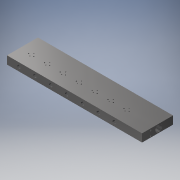
# Autodesk Inventor part: Ventilblock_4
Saved by Autodesk Inventor 2018 (Build 220112000, 112)
## iProperties
Created: 2011-11-24
Part Number: Ventilblock_4
Document SubType Name: Modeling
Designer: Neef
Density: 8 g/cm^3
Material: Stainless Steel
Appearance: Semi-Polished
Author: Neef
Autodesk Inventor part; units mm, degrees
ref_plane "YZ Plane" through (0, 0, 0) normal (1, 0, 0) x (0, 1, 0)
ref_plane "XZ Plane" through (0, 0, 0) normal (0, 1, 0) x (-1, 0, 0)
ref_plane "XY Plane" through (0, 0, 0) normal (0, 0, 1) x (1, 0, 0)
sketch "Skizze1" plane through (0, 0, 0) normal (0, 0, 1) x (1, 0, 0)
  line L0 (-85, 19.5) -> (85, 19.5)
  line L1 (85, 19.5) -> (85, -19.5)
  line L2 (85, -19.5) -> (-85, -19.5)
  line L3 (-85, -19.5) -> (-85, 19.5)
  line L4 (0, 27.3) -> (0, -27.3) projected
  line L5 (-119, 0) -> (119, 0) projected
  point P0 (0, 19.5)
  point P1 (85, 0)
  dimension "d0" = 39
  dimension "d1" = 170
  constraints: 8 end point, 2 midpoint, 2 parallel, 2 point on line, 1 horizontal, 1 perpendicular
  measures "d0" distance of L0.end L1.end
  measures "d1" distance of L0.start L0.end
extrude "Extrusion1" add sketch "Skizze1" along normal blind 10
sketch "Skizze2" plane through (0, 0, 10) normal (0, 0, 1) x (1, 0, 0)
  line L0 (-85, 19.5) -> (85, 19.5) projected
  line L1 (-85, -19.5) -> (-85, 19.5) projected
  line L2 (-75, 17.5) -> (-65, 17.5) construction
  line L3 (-65, 17.5) -> (-65, -9.5) construction
  line L4 (-65, -9.5) -> (-75, -9.5) construction
  line L5 (-75, -9.5) -> (-75, 17.5) construction
  line L6 (-70, -9.5) -> (-70, -1.8624) construction
  point P0 (-70, -0.7)
  point P1 (-70, -5.7)
  dimension "d6" = 10
  dimension "d7" = 27
  dimension "d8" = 5
  dimension "d9" = 10
  dimension "d10" = 3.8
  dimension "d11" = 2
  dimension "d12" = 5
  constraints: 10 end point, 2 parallel, 2 point on line, 1 horizontal, 1 midpoint, 1 perpendicular, 1 vertical
  measures "d6" distance of L2.start L2.end
  measures "d7" distance of L4.end L2.start
  measures "d8" distance between parallel lines of L3 L6
  measures "d9" distance between parallel lines of L5 L1
  measures "d10" distance from line of point (-70, -5.7) L4
  measures "d11" distance between parallel lines of L0 L2
  measures "d12" distance of point (-70, -5.7) point (-70, -0.7)
hole "Bohrung1" at (-70, -0.7, 10) at (-70, -5.7, 10) direction (0, 0, -1) diameter 1.2 depth 5 tip angle 118
sketch "Skizze3" plane through (0, 0, 10) normal (0, 0, 1) x (1, 0, 0)
  circle A0 centre (-70, -5.7) radius 0.6 projected
  circle A1 centre (-70, -0.7) radius 0.6 projected
  point P0 (-73.25, -4)
  point P1 (-66.75, -4)
  dimension "d20" = 3.25
  dimension "d21" = 3.25
  dimension "d22" = 1.7
  dimension "d23" = 1.7
  measures "d20" horizontal distance of A1.centre point (-66.75, -4)
  measures "d21" horizontal distance of A1.centre point (-73.25, -4)
  measures "d22" vertical distance of point (-66.75, -4) A0.centre
  measures "d23" vertical distance of A0.centre point (-73.25, -4)
hole "Bohrung2" at (-73.25, -4, 10) at (-66.75, -4, 10) direction (0, 0, -1) diameter 1.221 depth 7 tip angle 118 thread size "M1.6x0.35" class "6H" standard "ISO Metric profile"
pattern_linear "Rechteckige Anordnung1" count 7 spacing 20 along (1, 0, 0) of "Bohrung1", "Bohrung2"
sketch "Skizze5" plane through (-85, -19.5, 0) normal (0, -1, 0) x (1, 0, 0)
  line L0 (170, 10) -> (0, 10) projected
  line L1 (0, 0) -> (0, 10) projected
  line L2 (15.6, 5) -> (15.6, 10) projected
  line L3 (15.6, 5) -> (14.4, 5) projected
  line L4 (14.4, 5) -> (14.4, 10) projected
  point P0 (15, 5)
  dimension "d53" = 15
  dimension "d54" = 5
  constraints: 1 midpoint
  measures "d53" distance from line of L1 point (15, 5)
  measures "d54" distance from line of L0 point (15, 5)
hole "Bohrung5" at (-70, -19.5, 5) direction (0, 1, 0) diameter 2 depth 14 tip angle 118
hole "Bohrung6" at (-70, -19.5, 5) direction (0, 1, 0) diameter 4.134 depth 7 tip angle 118 thread size "M5x0.8" class "6H" standard "ISO Metric profile"
pattern_linear "Rechteckige Anordnung2" count 7 spacing 20 along (1, 0, 0) of "Bohrung5", "Bohrung6"
sketch "Skizze8" plane through (-85, -19.5, 0) normal (-1, 0, 0) x (0, 0, 1)
  line L0 (10, 0) -> (10, 39) projected
  line L1 (0, 39) -> (10, 39) projected
  line L2 (0, 0) -> (0, 39) projected
  point P0 (0, 19.5)
  point P1 (2, 11)
  point P2 (8, 11)
  dimension "d145" = 28
  dimension "d146" = 28
  dimension "d147" = 2
  dimension "d148" = 2
  measures "d145" distance from line of L1 point (8, 11)
  measures "d146" distance from line of L1 point (2, 11)
  measures "d147" distance from line of L0 point (8, 11)
  measures "d148" distance from line of L2 point (2, 11)
hole "Bohrung14" at (-85, -8.5, 2) at (-85, -8.5, 8) direction (1, 0, 0) diameter 2.459 depth 12 tip angle 118 thread size "M3x0.5" class "6H" standard "ISO Metric profile"
sketch "Skizze9" plane through (85, -19.5, 0) normal (1, 0, 0) x (0, 0, -1)
  circle A0 centre (-8, 11) radius 1.2295 projected
  circle A1 centre (-2, 11) radius 1.2295 projected
  point P0 (0, 19.5)
  constraints: 2 coincident
hole "Bohrung15" at (85, -8.5, 8) at (85, -8.5, 2) direction (-1, 0, 0) diameter 2.459 depth 12 tip angle 118 thread size "M3x0.5" class "6H" standard "ISO Metric profile"
sketch "Skizze10" plane through (85, -19.5, 0) normal (1, 0, 0) x (0, 0, -1)
  line L0 (0, 39) -> (-10, 39) projected
  circle A0 centre (-5, 21) radius 4 construction
  point P0 (0, 19.5)
  dimension "d163" = 18
  dimension "d164" = 8
  constraints: 1 centre point, 1 coincident
  measures "d163" distance from line of L0 point (-5, 21)
  measures "d164" diameter of A0
hole "Bohrung16" at (85, 1.5, 5) direction (-1, 0, 0) diameter 8 depth 166 tip angle 135
hole "Bohrung17" at (85, 1.5, 5) direction (-1, 0, 0) diameter 8.6 depth 12 tip angle 135
thread "Thread1" size "G9.728x0.907" designation "G 1/8" standard "JIS Pipe Threads" full length
equation "\"d21\" = d20"
equation "\"d23\" = d22"
equation "\"d146\" = d145"
equation "\"d148\" = d147"
